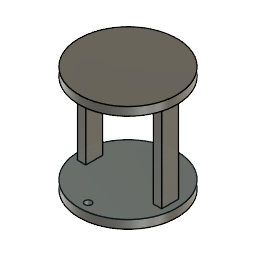
SEDS rocket av holder (Autodesk Fusion 360 design; units mm, degrees)
part number: 2026-05-26-13-21-48-249
Autodesk Fusion 360 part; units mm, degrees
sketch "Sketch1" plane through (0, 0, 0) normal (0, 0, 1) x (1, 0, 0)
  circle A0 centre (0, 0) radius 14
  dimension "d1" = 28
  constraint coincident A0.centre origin
  measures "d1" diameter of A0
sketch "Sketch2" plane through (0, 0, 0) normal (0, 0, 1) x (1, 0, 0)
sketch "Sketch3" plane through (0, 0, 4) normal (0, 0, 1) x (-1, 0, 0)
sketch "Sketch4" plane through (0, 0, 0) normal (0, 0, 1) x (1, 0, 0)
sketch "Sketch5" plane through (0, 0, 0) normal (0, 0, 1) x (1, 0, 0)
sketch "Sketch6" plane through (0, 0, 0) normal (0, 0, 1) x (1, 0, 0)
  circle A0 centre (0, 0) radius 29
  dimension "d9" = 58
  constraint coincident A0.centre origin
  measures "d9" diameter of A0
sketch "Sketch7" plane through (0, 0, 5) normal (0, 0, 1) x (-1, 0, 0)
  circle A0 centre (0, 0) radius 29
  circle A1 centre (0, -21) radius 2
  circle A2 centre (0, 21) radius 2
  dimension "d12" = 4
  dimension "d13" = 4
  measures "d12" diameter of A1
  measures "d13" diameter of A2
sketch "Sketch8" plane through (0, 0, 5) normal (0, 0, 1) x (1, 0, 0)
sketch "Sketch9" plane through (0, 0, 5) normal (0, 0, 1) x (-1, 0, 0)
  circle A0 centre (0, -21) radius 2
  circle A1 centre (0, 0) radius 29
  circle A2 centre (0, 24.215) radius 2
sketch "Sketch10" plane through (0, 0, 0) normal (0, 0, 1) x (1, 0, 0)
sketch "Sketch11" plane through (0, 0, 0) normal (0, 0, 1) x (1, 0, 0)
sketch "Sketch12" plane through (0, 0, 0) normal (0, 0, 1) x (1, 0, 0)
  circle A0 centre (0, 0) radius 29
  dimension "d18" = 58
  constraint coincident A0.centre origin
  measures "d18" diameter of A0
sketch "Sketch13" plane through (0, 0, 5) normal (0, 0, 1) x (-1, 0, 0)
  circle A0 centre (0, 0) radius 29
  circle A1 centre (0, -22) radius 2
  circle A2 centre (0, 23.212) radius 2
  dimension "d21" = 4
  dimension "d22" = 4
  dimension "d23" = 58
  dimension "d24" = 45.212
  measures "d21" diameter of A1
  measures "d22" diameter of A2
  measures "d23" diameter of A0
  measures "d24" distance of A1.centre A2.centre
sketch "Sketch14" plane through (0, 0, 5) normal (0, 0, 1) x (-1, 0, 0)
sketch "Sketch15" plane through (0, 0, 0) normal (0, 0, 1) x (1, 0, 0)
  circle A0 centre (0, 0) radius 29
  circle A1 centre (0, -23.666) radius 2
  line L0 (-25, -29) -> (20, -29)
  circle A2 centre (0, 21.546) radius 2
  dimension "d33" = 58
  dimension "d34" = 4
  dimension "d35" = 5.334
  dimension "d36" = 4
  constraint coincident A0.centre origin
  constraint horizontal L0
  measures "d33" diameter of A0
  measures "d34" diameter of A1
  measures "d35" distance of A1.centre L0
  measures "d36" diameter of A2
extrude "Extrude7" add sketch "Sketch15" along normal blind 5 makes body 1
sketch "Sketch16" plane through (0, 0, 5) normal (0, 0, 1) x (-1, 0, 0)
  circle A0 centre (0, -21.546) radius 2
  circle A1 centre (0, 23.666) radius 2
  circle A2 centre (0, 0) radius 29
  line L0 (25, -5) -> (20, -5)
  line L1 (20, -5) -> (20, 5)
  line L2 (20, 5) -> (25, 5)
  line L3 (25, 5) -> (25, -5)
  line L4 (-25, -5) -> (-20, -5)
  line L5 (-20, -5) -> (-20, 5)
  line L6 (-20, 5) -> (-25, 5)
  line L7 (-25, 5) -> (-25, -5)
  constraint horizontal L0
  constraint vertical L1
  constraint horizontal L2
  constraint vertical L3
  constraint horizontal L4
  constraint vertical L5
  constraint horizontal L6
  constraint vertical L7
extrude "Extrude8" add sketch "Sketch16" along normal blind 50 contours L0 L1 L2 L3 | L4 L5 L6 L7 bodies 1
sketch "Sketch17" plane through (0, 0, 5) normal (0, 0, 1) x (-1, 0, 0)
  line L0 (-25, 5) -> (-20, 5)
  line L1 (-20, 5) -> (-20, -5)
  line L2 (-20, -5) -> (-25, -5)
  line L3 (-25, -5) -> (-25, 5)
  line L4 (25, 5) -> (25, -5)
  line L5 (25, -5) -> (20, -5)
  line L6 (20, -5) -> (20, 5)
  line L7 (20, 5) -> (25, 5)
  circle A0 centre (0, -21.546) radius 2
  circle A1 centre (0, 23.666) radius 2
  circle A2 centre (0, 0) radius 29
sketch "Sketch18" plane through (0, 0, 55) normal (0, 0, 1) x (-1, 0, 0)
  line L0 (25, 5) -> (20, 5)
  line L1 (20, 5) -> (20, -5)
  line L2 (20, -5) -> (25, -5)
  line L3 (25, -5) -> (25, 5)
  line L4 (-20, 5) -> (-20, -5)
  dimension "d41" = 40
  measures "d41" distance of L1 L4
extrude "Extrude9" add sketch "Sketch18" 1 faces at (23.3333, 1.6667, 55) along normal blind 3 on bodies 1 bodies 1
sketch "Sketch19" plane through (0, 0, 58) normal (0, 0, 1) x (-1, 0, 0)
  line L0 (25, -5) -> (25, 5)
  line L1 (25, 5) -> (20, 5)
  line L2 (20, 5) -> (20, -5)
  line L3 (20, -5) -> (25, -5)
  line L4 (-20, 5) -> (-20, -5)
  circle A0 centre (0, 0) radius 29
  dimension "d44" = 40
  constraint coincident A0.centre origin
  measures "d44" distance of L2 L4
extrude "Extrude10" add sketch "Sketch19" along normal blind 5 separate body makes body 2
extrude "Extrude11" add 1 faces at (-21.6667, 1.6667, 58) along direction (0, 0, 1) blind 5 on bodies 1 bodies 1 2
sketch "Sketch20" plane through (0, 0, 0) normal (1, 0, 0) x (0, 1, 0)
sketch "Sketch21" plane through (0, 0, 0) normal (1, 0, 0) x (0, 1, 0)
